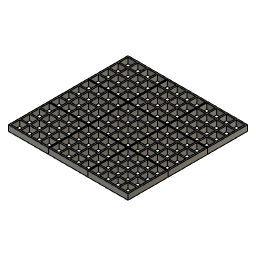
noycebru ws2812b 30 led per meter diffuser (Autodesk Fusion 360 design; units mm, degrees)
Autodesk Fusion 360 part; units mm, degrees
note: some values were not read from the file. Chosen so that the rebuilt part matches the saved one: which bodies a step acts on.
(part 1 of 2)
sketch "Sketch1" plane through (0, 0, 0) normal (0, 0, 1) x (1, 0, 0)
  line L0 (7.62, 66.04) -> (36.195, 66.04)
  line L1 (36.195, 66.04) -> (36.195, 37.465)
  line L2 (36.195, 37.465) -> (7.62, 37.465)
  line L3 (7.62, 37.465) -> (7.62, 66.04)
  line L4 (69.5325, 66.04) -> (69.5325, 37.465)
  line L5 (40.9575, 37.465) -> (40.9575, 66.04)
  line L6 (40.9575, 66.04) -> (69.5325, 66.04)
  line L7 (69.5325, 37.465) -> (40.9575, 37.465)
  line L8 (102.87, 66.04) -> (102.87, 37.465)
  line L9 (74.295, 37.465) -> (74.295, 66.04)
  line L10 (74.295, 66.04) -> (102.87, 66.04)
  line L11 (102.87, 37.465) -> (74.295, 37.465)
  line L12 (136.2075, 66.04) -> (136.2075, 37.465)
  line L13 (107.6325, 37.465) -> (107.6325, 66.04)
  line L14 (107.6325, 66.04) -> (136.2075, 66.04)
  line L15 (136.2075, 37.465) -> (107.6325, 37.465)
  line L16 (169.545, 66.04) -> (169.545, 37.465)
  line L17 (140.97, 37.465) -> (140.97, 66.04)
  line L18 (140.97, 66.04) -> (169.545, 66.04)
  line L19 (169.545, 37.465) -> (140.97, 37.465)
  line L20 (202.8825, 66.04) -> (202.8825, 37.465)
  line L21 (174.3075, 37.465) -> (174.3075, 66.04)
  line L22 (174.3075, 66.04) -> (202.8825, 66.04)
  line L23 (202.8825, 37.465) -> (174.3075, 37.465)
  line L24 (236.22, 66.04) -> (236.22, 37.465)
  line L25 (207.645, 37.465) -> (207.645, 66.04)
  line L26 (207.645, 66.04) -> (236.22, 66.04)
  line L27 (236.22, 37.465) -> (207.645, 37.465)
  line L28 (269.5575, 66.04) -> (269.5575, 37.465)
  line L29 (240.9825, 37.465) -> (240.9825, 66.04)
  line L30 (240.9825, 66.04) -> (269.5575, 66.04)
  line L31 (269.5575, 37.465) -> (240.9825, 37.465)
  line L32 (302.895, 66.04) -> (302.895, 37.465)
  line L33 (274.32, 37.465) -> (274.32, 66.04)
  line L34 (274.32, 66.04) -> (302.895, 66.04)
  line L35 (302.895, 37.465) -> (274.32, 37.465)
  line L36 (336.2325, 66.04) -> (336.2325, 37.465)
  line L37 (307.6575, 37.465) -> (307.6575, 66.04)
  line L38 (307.6575, 66.04) -> (336.2325, 66.04)
  line L39 (336.2325, 37.465) -> (307.6575, 37.465)
  line L40 (369.57, 66.04) -> (369.57, 37.465)
  line L41 (340.995, 37.465) -> (340.995, 66.04)
  line L42 (340.995, 66.04) -> (369.57, 66.04)
  line L43 (369.57, 37.465) -> (340.995, 37.465)
  line L44 (402.9075, 66.04) -> (402.9075, 37.465)
  line L45 (374.3325, 37.465) -> (374.3325, 66.04)
  line L46 (374.3325, 66.04) -> (402.9075, 66.04)
  line L47 (402.9075, 37.465) -> (374.3325, 37.465)
  line L48 (36.195, 99.3775) -> (36.195, 70.8025)
  line L49 (7.62, 70.8025) -> (7.62, 99.3775)
  line L50 (7.62, 99.3775) -> (36.195, 99.3775)
  line L51 (36.195, 70.8025) -> (7.62, 70.8025)
  line L52 (69.5325, 99.3775) -> (69.5325, 70.8025)
  line L53 (40.9575, 70.8025) -> (40.9575, 99.3775)
  line L54 (40.9575, 99.3775) -> (69.5325, 99.3775)
  line L55 (69.5325, 70.8025) -> (40.9575, 70.8025)
  line L56 (102.87, 99.3775) -> (102.87, 70.8025)
  line L57 (74.295, 70.8025) -> (74.295, 99.3775)
  line L58 (74.295, 99.3775) -> (102.87, 99.3775)
  line L59 (102.87, 70.8025) -> (74.295, 70.8025)
  line L60 (136.2075, 99.3775) -> (136.2075, 70.8025)
  line L61 (107.6325, 70.8025) -> (107.6325, 99.3775)
  line L62 (107.6325, 99.3775) -> (136.2075, 99.3775)
  line L63 (136.2075, 70.8025) -> (107.6325, 70.8025)
  line L64 (169.545, 99.3775) -> (169.545, 70.8025)
  line L65 (140.97, 70.8025) -> (140.97, 99.3775)
  line L66 (140.97, 99.3775) -> (169.545, 99.3775)
  line L67 (169.545, 70.8025) -> (140.97, 70.8025)
  line L68 (202.8825, 99.3775) -> (202.8825, 70.8025)
  line L69 (174.3075, 70.8025) -> (174.3075, 99.3775)
  line L70 (174.3075, 99.3775) -> (202.8825, 99.3775)
  line L71 (202.8825, 70.8025) -> (174.3075, 70.8025)
  line L72 (236.22, 99.3775) -> (236.22, 70.8025)
  line L73 (207.645, 70.8025) -> (207.645, 99.3775)
  line L74 (207.645, 99.3775) -> (236.22, 99.3775)
  line L75 (236.22, 70.8025) -> (207.645, 70.8025)
  line L76 (269.5575, 99.3775) -> (269.5575, 70.8025)
  line L77 (240.9825, 70.8025) -> (240.9825, 99.3775)
  line L78 (240.9825, 99.3775) -> (269.5575, 99.3775)
  line L79 (269.5575, 70.8025) -> (240.9825, 70.8025)
  line L80 (302.895, 99.3775) -> (302.895, 70.8025)
  line L81 (274.32, 70.8025) -> (274.32, 99.3775)
  line L82 (274.32, 99.3775) -> (302.895, 99.3775)
  line L83 (302.895, 70.8025) -> (274.32, 70.8025)
  line L84 (336.2325, 99.3775) -> (336.2325, 70.8025)
  line L85 (307.6575, 70.8025) -> (307.6575, 99.3775)
  line L86 (307.6575, 99.3775) -> (336.2325, 99.3775)
  line L87 (336.2325, 70.8025) -> (307.6575, 70.8025)
  line L88 (369.57, 99.3775) -> (369.57, 70.8025)
  line L89 (340.995, 70.8025) -> (340.995, 99.3775)
  line L90 (340.995, 99.3775) -> (369.57, 99.3775)
  line L91 (369.57, 70.8025) -> (340.995, 70.8025)
  line L92 (402.9075, 99.3775) -> (402.9075, 70.8025)
  line L93 (374.3325, 70.8025) -> (374.3325, 99.3775)
  line L94 (374.3325, 99.3775) -> (402.9075, 99.3775)
  line L95 (402.9075, 70.8025) -> (374.3325, 70.8025)
  line L96 (36.195, 132.715) -> (36.195, 104.14)
  line L97 (7.62, 104.14) -> (7.62, 132.715)
  line L98 (7.62, 132.715) -> (36.195, 132.715)
  line L99 (36.195, 104.14) -> (7.62, 104.14)
  line L100 (69.5325, 132.715) -> (69.5325, 104.14)
  line L101 (40.9575, 104.14) -> (40.9575, 132.715)
  line L102 (40.9575, 132.715) -> (69.5325, 132.715)
  line L103 (69.5325, 104.14) -> (40.9575, 104.14)
  line L104 (102.87, 132.715) -> (102.87, 104.14)
  line L105 (74.295, 104.14) -> (74.295, 132.715)
  line L106 (74.295, 132.715) -> (102.87, 132.715)
  line L107 (102.87, 104.14) -> (74.295, 104.14)
  line L108 (136.2075, 132.715) -> (136.2075, 104.14)
  line L109 (107.6325, 104.14) -> (107.6325, 132.715)
  line L110 (107.6325, 132.715) -> (136.2075, 132.715)
  line L111 (136.2075, 104.14) -> (107.6325, 104.14)
  line L112 (169.545, 132.715) -> (169.545, 104.14)
  line L113 (140.97, 104.14) -> (140.97, 132.715)
  line L114 (140.97, 132.715) -> (169.545, 132.715)
  line L115 (169.545, 104.14) -> (140.97, 104.14)
  line L116 (202.8825, 132.715) -> (202.8825, 104.14)
  line L117 (174.3075, 104.14) -> (174.3075, 132.715)
  line L118 (174.3075, 132.715) -> (202.8825, 132.715)
  line L119 (202.8825, 104.14) -> (174.3075, 104.14)
  line L120 (236.22, 132.715) -> (236.22, 104.14)
  line L121 (207.645, 104.14) -> (207.645, 132.715)
  line L122 (207.645, 132.715) -> (236.22, 132.715)
  line L123 (236.22, 104.14) -> (207.645, 104.14)
  line L124 (269.5575, 132.715) -> (269.5575, 104.14)
  line L125 (240.9825, 104.14) -> (240.9825, 132.715)
  line L126 (240.9825, 132.715) -> (269.5575, 132.715)
  line L127 (269.5575, 104.14) -> (240.9825, 104.14)
  line L128 (302.895, 132.715) -> (302.895, 104.14)
  line L129 (274.32, 104.14) -> (274.32, 132.715)
  line L130 (274.32, 132.715) -> (302.895, 132.715)
  line L131 (302.895, 104.14) -> (274.32, 104.14)
  line L132 (336.2325, 132.715) -> (336.2325, 104.14)
  line L133 (307.6575, 104.14) -> (307.6575, 132.715)
  line L134 (307.6575, 132.715) -> (336.2325, 132.715)
  line L135 (336.2325, 104.14) -> (307.6575, 104.14)
  line L136 (369.57, 132.715) -> (369.57, 104.14)
  line L137 (340.995, 104.14) -> (340.995, 132.715)
  line L138 (340.995, 132.715) -> (369.57, 132.715)
  line L139 (369.57, 104.14) -> (340.995, 104.14)
  line L140 (402.9075, 132.715) -> (402.9075, 104.14)
  line L141 (374.3325, 104.14) -> (374.3325, 132.715)
  line L142 (374.3325, 132.715) -> (402.9075, 132.715)
  line L143 (402.9075, 104.14) -> (374.3325, 104.14)
  line L144 (36.195, 166.0525) -> (36.195, 137.4775)
  line L145 (7.62, 137.4775) -> (7.62, 166.0525)
  line L146 (7.62, 166.0525) -> (36.195, 166.0525)
  line L147 (36.195, 137.4775) -> (7.62, 137.4775)
  line L148 (69.5325, 166.0525) -> (69.5325, 137.4775)
  line L149 (40.9575, 137.4775) -> (40.9575, 166.0525)
  line L150 (40.9575, 166.0525) -> (69.5325, 166.0525)
  line L151 (69.5325, 137.4775) -> (40.9575, 137.4775)
  line L152 (102.87, 166.0525) -> (102.87, 137.4775)
  line L153 (74.295, 137.4775) -> (74.295, 166.0525)
  line L154 (74.295, 166.0525) -> (102.87, 166.0525)
  line L155 (102.87, 137.4775) -> (74.295, 137.4775)
  line L156 (136.2075, 166.0525) -> (136.2075, 137.4775)
  line L157 (107.6325, 137.4775) -> (107.6325, 166.0525)
  line L158 (107.6325, 166.0525) -> (136.2075, 166.0525)
  line L159 (136.2075, 137.4775) -> (107.6325, 137.4775)
  line L160 (169.545, 166.0525) -> (169.545, 137.4775)
  line L161 (140.97, 137.4775) -> (140.97, 166.0525)
  line L162 (140.97, 166.0525) -> (169.545, 166.0525)
  line L163 (169.545, 137.4775) -> (140.97, 137.4775)
  line L164 (202.8825, 166.0525) -> (202.8825, 137.4775)
  line L165 (174.3075, 137.4775) -> (174.3075, 166.0525)
  line L166 (174.3075, 166.0525) -> (202.8825, 166.0525)
  line L167 (202.8825, 137.4775) -> (174.3075, 137.4775)
  line L168 (236.22, 166.0525) -> (236.22, 137.4775)
  line L169 (207.645, 137.4775) -> (207.645, 166.0525)
  line L170 (207.645, 166.0525) -> (236.22, 166.0525)
  line L171 (236.22, 137.4775) -> (207.645, 137.4775)
  line L172 (269.5575, 166.0525) -> (269.5575, 137.4775)
  line L173 (240.9825, 137.4775) -> (240.9825, 166.0525)
  line L174 (240.9825, 166.0525) -> (269.5575, 166.0525)
  line L175 (269.5575, 137.4775) -> (240.9825, 137.4775)
  line L176 (302.895, 166.0525) -> (302.895, 137.4775)
  line L177 (274.32, 137.4775) -> (274.32, 166.0525)
  line L178 (274.32, 166.0525) -> (302.895, 166.0525)
  line L179 (302.895, 137.4775) -> (274.32, 137.4775)
  line L180 (336.2325, 166.0525) -> (336.2325, 137.4775)
  line L181 (307.6575, 137.4775) -> (307.6575, 166.0525)
  line L182 (307.6575, 166.0525) -> (336.2325, 166.0525)
  line L183 (336.2325, 137.4775) -> (307.6575, 137.4775)
  line L184 (369.57, 166.0525) -> (369.57, 137.4775)
  line L185 (340.995, 137.4775) -> (340.995, 166.0525)
  line L186 (340.995, 166.0525) -> (369.57, 166.0525)
  line L187 (369.57, 137.4775) -> (340.995, 137.4775)
  line L188 (402.9075, 166.0525) -> (402.9075, 137.4775)
  line L189 (374.3325, 137.4775) -> (374.3325, 166.0525)
  line L190 (374.3325, 166.0525) -> (402.9075, 166.0525)
  line L191 (402.9075, 137.4775) -> (374.3325, 137.4775)
  line L192 (36.195, 199.39) -> (36.195, 170.815)
  line L193 (7.62, 170.815) -> (7.62, 199.39)
  line L194 (7.62, 199.39) -> (36.195, 199.39)
  line L195 (36.195, 170.815) -> (7.62, 170.815)
  line L196 (69.5325, 199.39) -> (69.5325, 170.815)
  line L197 (40.9575, 170.815) -> (40.9575, 199.39)
  line L198 (40.9575, 199.39) -> (69.5325, 199.39)
  line L199 (69.5325, 170.815) -> (40.9575, 170.815)
  line L200 (102.87, 199.39) -> (102.87, 170.815)
  line L201 (74.295, 170.815) -> (74.295, 199.39)
  line L202 (74.295, 199.39) -> (102.87, 199.39)
  line L203 (102.87, 170.815) -> (74.295, 170.815)
  line L204 (136.2075, 199.39) -> (136.2075, 170.815)
  line L205 (107.6325, 170.815) -> (107.6325, 199.39)
  line L206 (107.6325, 199.39) -> (136.2075, 199.39)
  line L207 (136.2075, 170.815) -> (107.6325, 170.815)
  line L208 (169.545, 199.39) -> (169.545, 170.815)
  line L209 (140.97, 170.815) -> (140.97, 199.39)
  line L210 (140.97, 199.39) -> (169.545, 199.39)
  line L211 (169.545, 170.815) -> (140.97, 170.815)
  line L212 (202.8825, 199.39) -> (202.8825, 170.815)
  line L213 (174.3075, 170.815) -> (174.3075, 199.39)
  line L214 (174.3075, 199.39) -> (202.8825, 199.39)
  line L215 (202.8825, 170.815) -> (174.3075, 170.815)
  line L216 (236.22, 199.39) -> (236.22, 170.815)
  line L217 (207.645, 170.815) -> (207.645, 199.39)
  line L218 (207.645, 199.39) -> (236.22, 199.39)
  line L219 (236.22, 170.815) -> (207.645, 170.815)
  line L220 (269.5575, 199.39) -> (269.5575, 170.815)
  line L221 (240.9825, 170.815) -> (240.9825, 199.39)
  line L222 (240.9825, 199.39) -> (269.5575, 199.39)
  line L223 (269.5575, 170.815) -> (240.9825, 170.815)
  line L224 (302.895, 199.39) -> (302.895, 170.815)
  line L225 (274.32, 170.815) -> (274.32, 199.39)
  line L226 (274.32, 199.39) -> (302.895, 199.39)
  line L227 (302.895, 170.815) -> (274.32, 170.815)
  line L228 (336.2325, 199.39) -> (336.2325, 170.815)
  line L229 (307.6575, 170.815) -> (307.6575, 199.39)
  line L230 (307.6575, 199.39) -> (336.2325, 199.39)
  line L231 (336.2325, 170.815) -> (307.6575, 170.815)
  line L232 (369.57, 199.39) -> (369.57, 170.815)
  line L233 (340.995, 170.815) -> (340.995, 199.39)
  line L234 (340.995, 199.39) -> (369.57, 199.39)
  line L235 (369.57, 170.815) -> (340.995, 170.815)
  line L236 (402.9075, 199.39) -> (402.9075, 170.815)
  line L237 (374.3325, 170.815) -> (374.3325, 199.39)
  line L238 (374.3325, 199.39) -> (402.9075, 199.39)
  line L239 (402.9075, 170.815) -> (374.3325, 170.815)
  line L240 (36.195, 232.7275) -> (36.195, 204.1525)
  line L241 (7.62, 204.1525) -> (7.62, 232.7275)
  line L242 (7.62, 232.7275) -> (36.195, 232.7275)
  line L243 (36.195, 204.1525) -> (7.62, 204.1525)
  line L244 (69.5325, 232.7275) -> (69.5325, 204.1525)
  line L245 (40.9575, 204.1525) -> (40.9575, 232.7275)
  line L246 (40.9575, 232.7275) -> (69.5325, 232.7275)
  line L247 (69.5325, 204.1525) -> (40.9575, 204.1525)
  line L248 (102.87, 232.7275) -> (102.87, 204.1525)
  line L249 (74.295, 204.1525) -> (74.295, 232.7275)
  line L250 (74.295, 232.7275) -> (102.87, 232.7275)
  line L251 (102.87, 204.1525) -> (74.295, 204.1525)
  line L252 (136.2075, 232.7275) -> (136.2075, 204.1525)
  line L253 (107.6325, 204.1525) -> (107.6325, 232.7275)
  line L254 (107.6325, 232.7275) -> (136.2075, 232.7275)
  line L255 (136.2075, 204.1525) -> (107.6325, 204.1525)
  line L256 (169.545, 232.7275) -> (169.545, 204.1525)
  line L257 (140.97, 204.1525) -> (140.97, 232.7275)
  line L258 (140.97, 232.7275) -> (169.545, 232.7275)
  line L259 (169.545, 204.1525) -> (140.97, 204.1525)
  line L260 (202.8825, 232.7275) -> (202.8825, 204.1525)
  line L261 (174.3075, 204.1525) -> (174.3075, 232.7275)
  line L262 (174.3075, 232.7275) -> (202.8825, 232.7275)
  line L263 (202.8825, 204.1525) -> (174.3075, 204.1525)
  line L264 (236.22, 232.7275) -> (236.22, 204.1525)
  line L265 (207.645, 204.1525) -> (207.645, 232.7275)
  line L266 (207.645, 232.7275) -> (236.22, 232.7275)
  line L267 (236.22, 204.1525) -> (207.645, 204.1525)
  line L268 (269.5575, 232.7275) -> (269.5575, 204.1525)
  line L269 (240.9825, 204.1525) -> (240.9825, 232.7275)
  line L270 (240.9825, 232.7275) -> (269.5575, 232.7275)
  line L271 (269.5575, 204.1525) -> (240.9825, 204.1525)
  line L272 (302.895, 232.7275) -> (302.895, 204.1525)
  line L273 (274.32, 204.1525) -> (274.32, 232.7275)
  line L274 (274.32, 232.7275) -> (302.895, 232.7275)
  line L275 (302.895, 204.1525) -> (274.32, 204.1525)
  line L276 (336.2325, 232.7275) -> (336.2325, 204.1525)
  line L277 (307.6575, 204.1525) -> (307.6575, 232.7275)
  line L278 (307.6575, 232.7275) -> (336.2325, 232.7275)
  line L279 (336.2325, 204.1525) -> (307.6575, 204.1525)
  line L280 (369.57, 232.7275) -> (369.57, 204.1525)
  line L281 (340.995, 204.1525) -> (340.995, 232.7275)
  line L282 (340.995, 232.7275) -> (369.57, 232.7275)
  line L283 (369.57, 204.1525) -> (340.995, 204.1525)
  line L284 (402.9075, 232.7275) -> (402.9075, 204.1525)
  line L285 (374.3325, 204.1525) -> (374.3325, 232.7275)
  line L286 (374.3325, 232.7275) -> (402.9075, 232.7275)
  line L287 (402.9075, 204.1525) -> (374.3325, 204.1525)
  line L288 (36.195, 266.065) -> (36.195, 237.49)
  line L289 (7.62, 237.49) -> (7.62, 266.065)
  line L290 (7.62, 266.065) -> (36.195, 266.065)
  line L291 (36.195, 237.49) -> (7.62, 237.49)
  line L292 (69.5325, 266.065) -> (69.5325, 237.49)
  line L293 (40.9575, 237.49) -> (40.9575, 266.065)
  line L294 (40.9575, 266.065) -> (69.5325, 266.065)
  line L295 (69.5325, 237.49) -> (40.9575, 237.49)
  line L296 (102.87, 266.065) -> (102.87, 237.49)
  line L297 (74.295, 237.49) -> (74.295, 266.065)
  line L298 (74.295, 266.065) -> (102.87, 266.065)
  line L299 (102.87, 237.49) -> (74.295, 237.49)
  line L300 (136.2075, 266.065) -> (136.2075, 237.49)
  line L301 (107.6325, 237.49) -> (107.6325, 266.065)
  line L302 (107.6325, 266.065) -> (136.2075, 266.065)
  line L303 (136.2075, 237.49) -> (107.6325, 237.49)
  line L304 (169.545, 266.065) -> (169.545, 237.49)
  line L305 (140.97, 237.49) -> (140.97, 266.065)
  line L306 (140.97, 266.065) -> (169.545, 266.065)
  line L307 (169.545, 237.49) -> (140.97, 237.49)
  line L308 (202.8825, 266.065) -> (202.8825, 237.49)
  line L309 (174.3075, 237.49) -> (174.3075, 266.065)
  line L310 (174.3075, 266.065) -> (202.8825, 266.065)
  line L311 (202.8825, 237.49) -> (174.3075, 237.49)
  line L312 (236.22, 266.065) -> (236.22, 237.49)
  line L313 (207.645, 237.49) -> (207.645, 266.065)
  line L314 (207.645, 266.065) -> (236.22, 266.065)
  line L315 (236.22, 237.49) -> (207.645, 237.49)
  line L316 (269.5575, 266.065) -> (269.5575, 237.49)
  line L317 (240.9825, 237.49) -> (240.9825, 266.065)
  line L318 (240.9825, 266.065) -> (269.5575, 266.065)
  line L319 (269.5575, 237.49) -> (240.9825, 237.49)
  line L320 (302.895, 266.065) -> (302.895, 237.49)
  line L321 (274.32, 237.49) -> (274.32, 266.065)
  line L322 (274.32, 266.065) -> (302.895, 266.065)
  line L323 (302.895, 237.49) -> (274.32, 237.49)
  line L324 (336.2325, 266.065) -> (336.2325, 237.49)
  line L325 (307.6575, 237.49) -> (307.6575, 266.065)
  line L326 (307.6575, 266.065) -> (336.2325, 266.065)
  line L327 (336.2325, 237.49) -> (307.6575, 237.49)
  line L328 (369.57, 266.065) -> (369.57, 237.49)
  line L329 (340.995, 237.49) -> (340.995, 266.065)
  line L330 (340.995, 266.065) -> (369.57, 266.065)
  line L331 (369.57, 237.49) -> (340.995, 237.49)
  line L332 (402.9075, 266.065) -> (402.9075, 237.49)
  line L333 (374.3325, 237.49) -> (374.3325, 266.065)
  line L334 (374.3325, 266.065) -> (402.9075, 266.065)
  line L335 (402.9075, 237.49) -> (374.3325, 237.49)
  line L336 (36.195, 299.4025) -> (36.195, 270.8275)
  line L337 (7.62, 270.8275) -> (7.62, 299.4025)
  line L338 (7.62, 299.4025) -> (36.195, 299.4025)
  line L339 (36.195, 270.8275) -> (7.62, 270.8275)
  line L340 (69.5325, 299.4025) -> (69.5325, 270.8275)
  line L341 (40.9575, 270.8275) -> (40.9575, 299.4025)
  line L342 (40.9575, 299.4025) -> (69.5325, 299.4025)
  line L343 (69.5325, 270.8275) -> (40.9575, 270.8275)
  line L344 (102.87, 299.4025) -> (102.87, 270.8275)
  line L345 (74.295, 270.8275) -> (74.295, 299.4025)
  line L346 (74.295, 299.4025) -> (102.87, 299.4025)
  line L347 (102.87, 270.8275) -> (74.295, 270.8275)
  line L348 (136.2075, 299.4025) -> (136.2075, 270.8275)
  line L349 (107.6325, 270.8275) -> (107.6325, 299.4025)
  line L350 (107.6325, 299.4025) -> (136.2075, 299.4025)
  line L351 (136.2075, 270.8275) -> (107.6325, 270.8275)
  line L352 (169.545, 299.4025) -> (169.545, 270.8275)
  line L353 (140.97, 270.8275) -> (140.97, 299.4025)
  line L354 (140.97, 299.4025) -> (169.545, 299.4025)
  line L355 (169.545, 270.8275) -> (140.97, 270.8275)
  line L356 (202.8825, 299.4025) -> (202.8825, 270.8275)
  line L357 (174.3075, 270.8275) -> (174.3075, 299.4025)
  line L358 (174.3075, 299.4025) -> (202.8825, 299.4025)
  line L359 (202.8825, 270.8275) -> (174.3075, 270.8275)
  line L360 (236.22, 299.4025) -> (236.22, 270.8275)
  line L361 (207.645, 270.8275) -> (207.645, 299.4025)
  line L362 (207.645, 299.4025) -> (236.22, 299.4025)
  line L363 (236.22, 270.8275) -> (207.645, 270.8275)
  line L364 (269.5575, 299.4025) -> (269.5575, 270.8275)
  line L365 (240.9825, 270.8275) -> (240.9825, 299.4025)
  line L366 (240.9825, 299.4025) -> (269.5575, 299.4025)
  line L367 (269.5575, 270.8275) -> (240.9825, 270.8275)
  line L368 (302.895, 299.4025) -> (302.895, 270.8275)
  line L369 (274.32, 270.8275) -> (274.32, 299.4025)
  line L370 (274.32, 299.4025) -> (302.895, 299.4025)
  line L371 (302.895, 270.8275) -> (274.32, 270.8275)
  line L372 (336.2325, 299.4025) -> (336.2325, 270.8275)
  line L373 (307.6575, 270.8275) -> (307.6575, 299.4025)
  line L374 (307.6575, 299.4025) -> (336.2325, 299.4025)
  line L375 (336.2325, 270.8275) -> (307.6575, 270.8275)
  line L376 (369.57, 299.4025) -> (369.57, 270.8275)
  line L377 (340.995, 270.8275) -> (340.995, 299.4025)
  line L378 (340.995, 299.4025) -> (369.57, 299.4025)
  line L379 (369.57, 270.8275) -> (340.995, 270.8275)
  line L380 (402.9075, 299.4025) -> (402.9075, 270.8275)
  line L381 (374.3325, 270.8275) -> (374.3325, 299.4025)
  line L382 (374.3325, 299.4025) -> (402.9075, 299.4025)
  line L383 (402.9075, 270.8275) -> (374.3325, 270.8275)
  line L384 (36.195, 332.74) -> (36.195, 304.165)
  line L385 (7.62, 304.165) -> (7.62, 332.74)
  line L386 (7.62, 332.74) -> (36.195, 332.74)
  line L387 (36.195, 304.165) -> (7.62, 304.165)
  line L388 (69.5325, 332.74) -> (69.5325, 304.165)
  line L389 (40.9575, 304.165) -> (40.9575, 332.74)
  line L390 (40.9575, 332.74) -> (69.5325, 332.74)
  line L391 (69.5325, 304.165) -> (40.9575, 304.165)
  line L392 (102.87, 332.74) -> (102.87, 304.165)
  line L393 (74.295, 304.165) -> (74.295, 332.74)
  line L394 (74.295, 332.74) -> (102.87, 332.74)
  line L395 (102.87, 304.165) -> (74.295, 304.165)
  line L396 (136.2075, 332.74) -> (136.2075, 304.165)
  line L397 (107.6325, 304.165) -> (107.6325, 332.74)
  line L398 (107.6325, 332.74) -> (136.2075, 332.74)
  line L399 (136.2075, 304.165) -> (107.6325, 304.165)
  line L400 (169.545, 332.74) -> (169.545, 304.165)
  line L401 (140.97, 304.165) -> (140.97, 332.74)
  line L402 (140.97, 332.74) -> (169.545, 332.74)
  line L403 (169.545, 304.165) -> (140.97, 304.165)
  line L404 (202.8825, 332.74) -> (202.8825, 304.165)
  line L405 (174.3075, 304.165) -> (174.3075, 332.74)
  line L406 (174.3075, 332.74) -> (202.8825, 332.74)
  line L407 (202.8825, 304.165) -> (174.3075, 304.165)
  line L408 (236.22, 332.74) -> (236.22, 304.165)
  line L409 (207.645, 304.165) -> (207.645, 332.74)
  line L410 (207.645, 332.74) -> (236.22, 332.74)
  line L411 (236.22, 304.165) -> (207.645, 304.165)
  line L412 (269.5575, 332.74) -> (269.5575, 304.165)
  line L413 (240.9825, 304.165) -> (240.9825, 332.74)
  line L414 (240.9825, 332.74) -> (269.5575, 332.74)
  line L415 (269.5575, 304.165) -> (240.9825, 304.165)
  line L416 (302.895, 332.74) -> (302.895, 304.165)
  line L417 (274.32, 304.165) -> (274.32, 332.74)
  line L418 (274.32, 332.74) -> (302.895, 332.74)
  line L419 (302.895, 304.165) -> (274.32, 304.165)
  line L420 (336.2325, 332.74) -> (336.2325, 304.165)
  line L421 (307.6575, 304.165) -> (307.6575, 332.74)
  line L422 (307.6575, 332.74) -> (336.2325, 332.74)
  line L423 (336.2325, 304.165) -> (307.6575, 304.165)
  line L424 (369.57, 332.74) -> (369.57, 304.165)
  line L425 (340.995, 304.165) -> (340.995, 332.74)
  line L426 (340.995, 332.74) -> (369.57, 332.74)
  line L427 (369.57, 304.165) -> (340.995, 304.165)
  line L428 (402.9075, 332.74) -> (402.9075, 304.165)
  line L429 (374.3325, 304.165) -> (374.3325, 332.74)
  line L430 (374.3325, 332.74) -> (402.9075, 332.74)
  line L431 (402.9075, 304.165) -> (374.3325, 304.165)
  line L432 (36.195, 366.0775) -> (36.195, 337.5025)
  line L433 (7.62, 337.5025) -> (7.62, 366.0775)
  line L434 (7.62, 366.0775) -> (36.195, 366.0775)
  line L435 (36.195, 337.5025) -> (7.62, 337.5025)
  line L436 (69.5325, 366.0775) -> (69.5325, 337.5025)
  line L437 (40.9575, 337.5025) -> (40.9575, 366.0775)
  line L438 (40.9575, 366.0775) -> (69.5325, 366.0775)
  line L439 (69.5325, 337.5025) -> (40.9575, 337.5025)
  line L440 (102.87, 366.0775) -> (102.87, 337.5025)
  line L441 (74.295, 337.5025) -> (74.295, 366.0775)
  line L442 (74.295, 366.0775) -> (102.87, 366.0775)
  line L443 (102.87, 337.5025) -> (74.295, 337.5025)
  line L444 (136.2075, 366.0775) -> (136.2075, 337.5025)
  line L445 (107.6325, 337.5025) -> (107.6325, 366.0775)
  line L446 (107.6325, 366.0775) -> (136.2075, 366.0775)
  line L447 (136.2075, 337.5025) -> (107.6325, 337.5025)
  line L448 (169.545, 366.0775) -> (169.545, 337.5025)
  line L449 (140.97, 337.5025) -> (140.97, 366.0775)
  line L450 (140.97, 366.0775) -> (169.545, 366.0775)
  line L451 (169.545, 337.5025) -> (140.97, 337.5025)
  line L452 (202.8825, 366.0775) -> (202.8825, 337.5025)
  line L453 (174.3075, 337.5025) -> (174.3075, 366.0775)
  line L454 (174.3075, 366.0775) -> (202.8825, 366.0775)
  line L455 (202.8825, 337.5025) -> (174.3075, 337.5025)
  line L456 (236.22, 366.0775) -> (236.22, 337.5025)
  line L457 (207.645, 337.5025) -> (207.645, 366.0775)
  line L458 (207.645, 366.0775) -> (236.22, 366.0775)
  line L459 (236.22, 337.5025) -> (207.645, 337.5025)
  line L460 (269.5575, 366.0775) -> (269.5575, 337.5025)
  line L461 (240.9825, 337.5025) -> (240.9825, 366.0775)
  line L462 (240.9825, 366.0775) -> (269.5575, 366.0775)
  line L463 (269.5575, 337.5025) -> (240.9825, 337.5025)
  line L464 (302.895, 366.0775) -> (302.895, 337.5025)
  line L465 (274.32, 337.5025) -> (274.32, 366.0775)
  line L466 (274.32, 366.0775) -> (302.895, 366.0775)
  line L467 (302.895, 337.5025) -> (274.32, 337.5025)
  line L468 (336.2325, 366.0775) -> (336.2325, 337.5025)
  line L469 (307.6575, 337.5025) -> (307.6575, 366.0775)
  line L470 (307.6575, 366.0775) -> (336.2325, 366.0775)
  line L471 (336.2325, 337.5025) -> (307.6575, 337.5025)
  line L472 (369.57, 366.0775) -> (369.57, 337.5025)
  line L473 (340.995, 337.5025) -> (340.995, 366.0775)
  line L474 (340.995, 366.0775) -> (369.57, 366.0775)
  line L475 (369.57, 337.5025) -> (340.995, 337.5025)
  line L476 (402.9075, 366.0775) -> (402.9075, 337.5025)
  line L477 (374.3325, 337.5025) -> (374.3325, 366.0775)
  line L478 (374.3325, 366.0775) -> (402.9075, 366.0775)
  line L479 (402.9075, 337.5025) -> (374.3325, 337.5025)
  line L480 (36.195, 399.415) -> (36.195, 370.84)
  line L481 (7.62, 370.84) -> (7.62, 399.415)
  line L482 (7.62, 399.415) -> (36.195, 399.415)
  line L483 (36.195, 370.84) -> (7.62, 370.84)
  line L484 (69.5325, 399.415) -> (69.5325, 370.84)
  line L485 (40.9575, 370.84) -> (40.9575, 399.415)
  line L486 (40.9575, 399.415) -> (69.5325, 399.415)
  line L487 (69.5325, 370.84) -> (40.9575, 370.84)
  line L488 (102.87, 399.415) -> (102.87, 370.84)
  line L489 (74.295, 370.84) -> (74.295, 399.415)
  line L490 (74.295, 399.415) -> (102.87, 399.415)
  line L491 (102.87, 370.84) -> (74.295, 370.84)
  line L492 (136.2075, 399.415) -> (136.2075, 370.84)
  line L493 (107.6325, 370.84) -> (107.6325, 399.415)
  line L494 (107.6325, 399.415) -> (136.2075, 399.415)
  line L495 (136.2075, 370.84) -> (107.6325, 370.84)
  line L496 (169.545, 399.415) -> (169.545, 370.84)
  line L497 (140.97, 370.84) -> (140.97, 399.415)
  line L498 (140.97, 399.415) -> (169.545, 399.415)
  line L499 (169.545, 370.84) -> (140.97, 370.84)
  line L500 (202.8825, 399.415) -> (202.8825, 370.84)
  line L501 (174.3075, 370.84) -> (174.3075, 399.415)
  line L502 (174.3075, 399.415) -> (202.8825, 399.415)
  line L503 (202.8825, 370.84) -> (174.3075, 370.84)
  line L504 (236.22, 399.415) -> (236.22, 370.84)
  line L505 (207.645, 370.84) -> (207.645, 399.415)
  line L506 (207.645, 399.415) -> (236.22, 399.415)
  line L507 (236.22, 370.84) -> (207.645, 370.84)
  line L508 (269.5575, 399.415) -> (269.5575, 370.84)
  line L509 (240.9825, 370.84) -> (240.9825, 399.415)
  line L510 (240.9825, 399.415) -> (269.5575, 399.415)
  line L511 (269.5575, 370.84) -> (240.9825, 370.84)
  line L512 (302.895, 399.415) -> (302.895, 370.84)
  line L513 (274.32, 370.84) -> (274.32, 399.415)
  line L514 (274.32, 399.415) -> (302.895, 399.415)
  line L515 (302.895, 370.84) -> (274.32, 370.84)
  line L516 (336.2325, 399.415) -> (336.2325, 370.84)
  line L517 (307.6575, 370.84) -> (307.6575, 399.415)
  line L518 (307.6575, 399.415) -> (336.2325, 399.415)
  line L519 (336.2325, 370.84) -> (307.6575, 370.84)
  line L520 (369.57, 399.415) -> (369.57, 370.84)
  line L521 (340.995, 370.84) -> (340.995, 399.415)
  line L522 (340.995, 399.415) -> (369.57, 399.415)
  line L523 (369.57, 370.84) -> (340.995, 370.84)
  line L524 (402.9075, 399.415) -> (402.9075, 370.84)
  line L525 (374.3325, 370.84) -> (374.3325, 399.415)
  line L526 (374.3325, 399.415) -> (402.9075, 399.415)
  line L527 (402.9075, 370.84) -> (374.3325, 370.84)
  line L528 (36.195, 432.7525) -> (36.195, 404.1775)
  line L529 (7.62, 404.1775) -> (7.62, 432.7525)
  line L530 (7.62, 432.7525) -> (36.195, 432.7525)
  line L531 (36.195, 404.1775) -> (7.62, 404.1775)
  line L532 (69.5325, 432.7525) -> (69.5325, 404.1775)
  line L533 (40.9575, 404.1775) -> (40.9575, 432.7525)
  line L534 (40.9575, 432.7525) -> (69.5325, 432.7525)
  line L535 (69.5325, 404.1775) -> (40.9575, 404.1775)
  line L536 (102.87, 432.7525) -> (102.87, 404.1775)
  line L537 (74.295, 404.1775) -> (74.295, 432.7525)
  line L538 (74.295, 432.7525) -> (102.87, 432.7525)
  line L539 (102.87, 404.1775) -> (74.295, 404.1775)
  line L540 (136.2075, 432.7525) -> (136.2075, 404.1775)
  line L541 (107.6325, 404.1775) -> (107.6325, 432.7525)
  line L542 (107.6325, 432.7525) -> (136.2075, 432.7525)
  line L543 (136.2075, 404.1775) -> (107.6325, 404.1775)
  line L544 (169.545, 432.7525) -> (169.545, 404.1775)
  line L545 (140.97, 404.1775) -> (140.97, 432.7525)
  line L546 (140.97, 432.7525) -> (169.545, 432.7525)
  line L547 (169.545, 404.1775) -> (140.97, 404.1775)
  line L548 (202.8825, 432.7525) -> (202.8825, 404.1775)
  line L549 (174.3075, 404.1775) -> (174.3075, 432.7525)
  line L550 (174.3075, 432.7525) -> (202.8825, 432.7525)
  line L551 (202.8825, 404.1775) -> (174.3075, 404.1775)
  line L552 (236.22, 432.7525) -> (236.22, 404.1775)
  line L553 (207.645, 404.1775) -> (207.645, 432.7525)
  line L554 (207.645, 432.7525) -> (236.22, 432.7525)
  line L555 (236.22, 404.1775) -> (207.645, 404.1775)
  line L556 (269.5575, 432.7525) -> (269.5575, 404.1775)
  line L557 (240.9825, 404.1775) -> (240.9825, 432.7525)
  line L558 (240.9825, 432.7525) -> (269.5575, 432.7525)
  line L559 (269.5575, 404.1775) -> (240.9825, 404.1775)
  line L560 (302.895, 432.7525) -> (302.895, 404.1775)
  line L561 (274.32, 404.1775) -> (274.32, 432.7525)
  line L562 (274.32, 432.7525) -> (302.895, 432.7525)
  line L563 (302.895, 404.1775) -> (274.32, 404.1775)
  line L564 (336.2325, 432.7525) -> (336.2325, 404.1775)
  line L565 (307.6575, 404.1775) -> (307.6575, 432.7525)
  line L566 (307.6575, 432.7525) -> (336.2325, 432.7525)
  line L567 (336.2325, 404.1775) -> (307.6575, 404.1775)
  line L568 (369.57, 432.7525) -> (369.57, 404.1775)
  line L569 (340.995, 404.1775) -> (340.995, 432.7525)
  line L570 (340.995, 432.7525) -> (369.57, 432.7525)
  line L571 (369.57, 404.1775) -> (340.995, 404.1775)
  line L572 (402.9075, 432.7525) -> (402.9075, 404.1775)
  line L573 (374.3325, 404.1775) -> (374.3325, 432.7525)
  line L574 (374.3325, 432.7525) -> (402.9075, 432.7525)
  line L575 (402.9075, 404.1775) -> (374.3325, 404.1775)
  line L576 (36.195, 399.415) -> (7.62, 399.415)
  line L577 (2.8575, 399.415) -> (2.8575, 437.515)
  line L578 (2.8575, 437.515) -> (40.9575, 437.515)
  line L579 (40.9575, 432.7525) -> (40.9575, 404.1775)
  line L580 (402.9075, 399.415) -> (374.3325, 399.415)
  line L581 (369.57, 404.1775) -> (369.57, 432.7525)
  line L582 (369.57, 437.515) -> (407.67, 437.515)
  line L583 (407.67, 437.515) -> (407.67, 399.415)
  line L584 (40.9575, 437.515) -> (369.57, 437.515)
  line L585 (369.57, 432.7525) -> (40.9575, 432.7525)
  line L586 (407.67, 32.7025) -> (369.57, 32.7025)
  line L587 (374.3325, 70.8025) -> (402.9075, 70.8025)
  line L588 (407.67, 70.8025) -> (407.67, 32.7025)
  line L589 (40.9575, 32.7025) -> (2.8575, 32.7025)
  line L590 (2.8575, 32.7025) -> (2.8575, 70.8025)
  line L591 (7.62, 70.8025) -> (36.195, 70.8025)
  line L592 (40.9575, 66.04) -> (40.9575, 37.465)
  line L593 (7.62, 399.415) -> (7.62, 70.8025)
  line L594 (2.8575, 70.8025) -> (2.8575, 399.415)
  line L595 (402.9075, 399.415) -> (402.9075, 70.8025)
  line L596 (407.67, 70.8025) -> (407.67, 399.415)
  line L597 (369.57, 32.7025) -> (40.9575, 32.7025)
  line L598 (40.9575, 37.465) -> (369.57, 37.465)
  dimension "d1" = 28.575
  dimension "d2" = 28.575
  dimension "d5" = 33.3375
  dimension "d6" = 33.3375
  constraint horizontal L0
  constraint vertical L1
  constraint horizontal L2
  constraint vertical L3
  constraint horizontal L584
  constraint horizontal L585
  constraint parallel L531 L576
  constraint parallel L529 L577
  constraint parallel L530 L578
  constraint parallel L528 L579
  constraint parallel L575 L580
  constraint parallel L573 L581
  constraint parallel L574 L582
  constraint parallel L572 L583
  constraint vertical L593
  constraint vertical L594
  constraint vertical L595
  constraint vertical L596
  constraint horizontal L597
  constraint horizontal L598
  constraint parallel L2 L589
  constraint parallel L3 L590
  constraint parallel L0 L591
  constraint parallel L1 L592
  constraint parallel L47 L586
  constraint parallel L46 L587
  constraint parallel L44 L588
  measures "d1" distance of L0.start L2.end
  measures "d2" distance of L0.start L0.end
extrude "Extrude1" add sketch "Sketch1" along normal blind 19.05 makes body 1
sketch "Sketch2" plane through (0, 0, 19.05) normal (0, 0, 1) x (-1, 0, 0)
  line L0 (-302.895, -132.715) -> (-302.895, -104.14)
  line L1 (-302.895, -104.14) -> (-274.32, -104.14)
  line L2 (-274.32, -104.14) -> (-274.32, -132.715)
  line L3 (-274.32, -132.715) -> (-302.895, -132.715)
  line L4 (-336.2325, -132.715) -> (-336.2325, -104.14)
  line L5 (-336.2325, -104.14) -> (-307.6575, -104.14)
  line L6 (-307.6575, -104.14) -> (-307.6575, -132.715)
  line L7 (-307.6575, -132.715) -> (-336.2325, -132.715)
  line L8 (-369.57, -132.715) -> (-369.57, -104.14)
  line L9 (-369.57, -104.14) -> (-340.995, -104.14)
  line L10 (-340.995, -104.14) -> (-340.995, -132.715)
  line L11 (-340.995, -132.715) -> (-369.57, -132.715)
  line L12 (-69.5325, -166.0525) -> (-69.5325, -137.4775)
  line L13 (-69.5325, -137.4775) -> (-40.9575, -137.4775)
  line L14 (-40.9575, -137.4775) -> (-40.9575, -166.0525)
  line L15 (-40.9575, -166.0525) -> (-69.5325, -166.0525)
  line L16 (-102.87, -166.0525) -> (-102.87, -137.4775)
  line L17 (-102.87, -137.4775) -> (-74.295, -137.4775)
  line L18 (-74.295, -137.4775) -> (-74.295, -166.0525)
  line L19 (-74.295, -166.0525) -> (-102.87, -166.0525)
  line L20 (-136.2075, -166.0525) -> (-136.2075, -137.4775)
  line L21 (-136.2075, -137.4775) -> (-107.6325, -137.4775)
  line L22 (-107.6325, -137.4775) -> (-107.6325, -166.0525)
  line L23 (-107.6325, -166.0525) -> (-136.2075, -166.0525)
  line L24 (-169.545, -166.0525) -> (-169.545, -137.4775)
  line L25 (-169.545, -137.4775) -> (-140.97, -137.4775)
  line L26 (-140.97, -137.4775) -> (-140.97, -166.0525)
  line L27 (-140.97, -166.0525) -> (-169.545, -166.0525)
  line L28 (-202.8825, -166.0525) -> (-202.8825, -137.4775)
  line L29 (-202.8825, -137.4775) -> (-174.3075, -137.4775)
  line L30 (-174.3075, -137.4775) -> (-174.3075, -166.0525)
  line L31 (-174.3075, -166.0525) -> (-202.8825, -166.0525)
  line L32 (-236.22, -166.0525) -> (-236.22, -137.4775)
  line L33 (-236.22, -137.4775) -> (-207.645, -137.4775)
  line L34 (-207.645, -137.4775) -> (-207.645, -166.0525)
  line L35 (-207.645, -166.0525) -> (-236.22, -166.0525)
  line L36 (-269.5575, -166.0525) -> (-269.5575, -137.4775)
  line L37 (-269.5575, -137.4775) -> (-240.9825, -137.4775)
  line L38 (-240.9825, -137.4775) -> (-240.9825, -166.0525)
  line L39 (-240.9825, -166.0525) -> (-269.5575, -166.0525)
  line L40 (-302.895, -166.0525) -> (-302.895, -137.4775)
  line L41 (-302.895, -137.4775) -> (-274.32, -137.4775)
  line L42 (-274.32, -137.4775) -> (-274.32, -166.0525)
  line L43 (-274.32, -166.0525) -> (-302.895, -166.0525)
  line L44 (-336.2325, -166.0525) -> (-336.2325, -137.4775)
  line L45 (-336.2325, -137.4775) -> (-307.6575, -137.4775)
  line L46 (-307.6575, -137.4775) -> (-307.6575, -166.0525)
  line L47 (-307.6575, -166.0525) -> (-336.2325, -166.0525)
  line L48 (-369.57, -166.0525) -> (-369.57, -137.4775)
  line L49 (-369.57, -137.4775) -> (-340.995, -137.4775)
  line L50 (-340.995, -137.4775) -> (-340.995, -166.0525)
  line L51 (-340.995, -166.0525) -> (-369.57, -166.0525)
  line L52 (-69.5325, -199.39) -> (-69.5325, -170.815)
  line L53 (-69.5325, -170.815) -> (-40.9575, -170.815)
  line L54 (-40.9575, -170.815) -> (-40.9575, -199.39)
  line L55 (-40.9575, -199.39) -> (-69.5325, -199.39)
  line L56 (-102.87, -199.39) -> (-102.87, -170.815)
  line L57 (-102.87, -170.815) -> (-74.295, -170.815)
  line L58 (-74.295, -170.815) -> (-74.295, -199.39)
  line L59 (-74.295, -199.39) -> (-102.87, -199.39)
  line L60 (-136.2075, -199.39) -> (-136.2075, -170.815)
  line L61 (-136.2075, -170.815) -> (-107.6325, -170.815)
  line L62 (-107.6325, -170.815) -> (-107.6325, -199.39)
  line L63 (-107.6325, -199.39) -> (-136.2075, -199.39)
  line L64 (-169.545, -199.39) -> (-169.545, -170.815)
  line L65 (-169.545, -170.815) -> (-140.97, -170.815)
  line L66 (-140.97, -170.815) -> (-140.97, -199.39)
  line L67 (-140.97, -199.39) -> (-169.545, -199.39)
  line L68 (-202.8825, -199.39) -> (-202.8825, -170.815)
  line L69 (-202.8825, -170.815) -> (-174.3075, -170.815)
  line L70 (-174.3075, -170.815) -> (-174.3075, -199.39)
  line L71 (-174.3075, -199.39) -> (-202.8825, -199.39)
  line L72 (-236.22, -199.39) -> (-236.22, -170.815)
  line L73 (-236.22, -170.815) -> (-207.645, -170.815)
  line L74 (-207.645, -170.815) -> (-207.645, -199.39)
  line L75 (-207.645, -199.39) -> (-236.22, -199.39)
  line L76 (-269.5575, -199.39) -> (-269.5575, -170.815)
  line L77 (-269.5575, -170.815) -> (-240.9825, -170.815)
  line L78 (-240.9825, -170.815) -> (-240.9825, -199.39)
  line L79 (-240.9825, -199.39) -> (-269.5575, -199.39)
  line L80 (-302.895, -199.39) -> (-302.895, -170.815)
  line L81 (-302.895, -170.815) -> (-274.32, -170.815)
  line L82 (-274.32, -170.815) -> (-274.32, -199.39)
  line L83 (-274.32, -199.39) -> (-302.895, -199.39)
  line L84 (-336.2325, -199.39) -> (-336.2325, -170.815)
  line L85 (-336.2325, -170.815) -> (-307.6575, -170.815)
  line L86 (-307.6575, -170.815) -> (-307.6575, -199.39)
  line L87 (-307.6575, -199.39) -> (-336.2325, -199.39)
  line L88 (-369.57, -199.39) -> (-369.57, -170.815)
  line L89 (-369.57, -170.815) -> (-340.995, -170.815)
  line L90 (-340.995, -170.815) -> (-340.995, -199.39)
  line L91 (-340.995, -199.39) -> (-369.57, -199.39)
  line L92 (-69.5325, -232.7275) -> (-69.5325, -204.1525)
  line L93 (-69.5325, -204.1525) -> (-40.9575, -204.1525)
  line L94 (-40.9575, -204.1525) -> (-40.9575, -232.7275)
  line L95 (-40.9575, -232.7275) -> (-69.5325, -232.7275)
  line L96 (-102.87, -232.7275) -> (-102.87, -204.1525)
  line L97 (-102.87, -204.1525) -> (-74.295, -204.1525)
  line L98 (-74.295, -204.1525) -> (-74.295, -232.7275)
  line L99 (-74.295, -232.7275) -> (-102.87, -232.7275)
  line L100 (-136.2075, -232.7275) -> (-136.2075, -204.1525)
  line L101 (-136.2075, -204.1525) -> (-107.6325, -204.1525)
  line L102 (-107.6325, -204.1525) -> (-107.6325, -232.7275)
  line L103 (-107.6325, -232.7275) -> (-136.2075, -232.7275)
  line L104 (-169.545, -232.7275) -> (-169.545, -204.1525)
  line L105 (-169.545, -204.1525) -> (-140.97, -204.1525)
  line L106 (-140.97, -204.1525) -> (-140.97, -232.7275)
  line L107 (-140.97, -232.7275) -> (-169.545, -232.7275)
  line L108 (-202.8825, -232.7275) -> (-202.8825, -204.1525)
  line L109 (-202.8825, -204.1525) -> (-174.3075, -204.1525)
  line L110 (-174.3075, -204.1525) -> (-174.3075, -232.7275)
  line L111 (-174.3075, -232.7275) -> (-202.8825, -232.7275)
  line L112 (-236.22, -232.7275) -> (-236.22, -204.1525)
  line L113 (-236.22, -204.1525) -> (-207.645, -204.1525)
  line L114 (-207.645, -204.1525) -> (-207.645, -232.7275)
  line L115 (-207.645, -232.7275) -> (-236.22, -232.7275)
  line L116 (-269.5575, -232.7275) -> (-269.5575, -204.1525)
  line L117 (-269.5575, -204.1525) -> (-240.9825, -204.1525)
  line L118 (-240.9825, -204.1525) -> (-240.9825, -232.7275)
  line L119 (-240.9825, -232.7275) -> (-269.5575, -232.7275)
  line L120 (-302.895, -232.7275) -> (-302.895, -204.1525)
  line L121 (-302.895, -204.1525) -> (-274.32, -204.1525)
  line L122 (-274.32, -204.1525) -> (-274.32, -232.7275)
  line L123 (-274.32, -232.7275) -> (-302.895, -232.7275)
  line L124 (-336.2325, -232.7275) -> (-336.2325, -204.1525)
  line L125 (-336.2325, -204.1525) -> (-307.6575, -204.1525)
  line L126 (-307.6575, -204.1525) -> (-307.6575, -232.7275)
  line L127 (-307.6575, -232.7275) -> (-336.2325, -232.7275)
  line L128 (-369.57, -232.7275) -> (-369.57, -204.1525)
  line L129 (-369.57, -204.1525) -> (-340.995, -204.1525)
  line L130 (-340.995, -204.1525) -> (-340.995, -232.7275)
  line L131 (-340.995, -232.7275) -> (-369.57, -232.7275)
  line L132 (-207.645, -432.7525) -> (-236.22, -432.7525)
  line L133 (-236.22, -432.7525) -> (-236.22, -404.1775)
  line L134 (-236.22, -404.1775) -> (-207.645, -404.1775)
  line L135 (-207.645, -404.1775) -> (-207.645, -432.7525)
  line L136 (-174.3075, -432.7525) -> (-202.8825, -432.7525)
  line L137 (-202.8825, -432.7525) -> (-202.8825, -404.1775)
  line L138 (-202.8825, -404.1775) -> (-174.3075, -404.1775)
  line L139 (-174.3075, -404.1775) -> (-174.3075, -432.7525)
  line L140 (-140.97, -432.7525) -> (-169.545, -432.7525)
  line L141 (-169.545, -432.7525) -> (-169.545, -404.1775)
  line L142 (-169.545, -404.1775) -> (-140.97, -404.1775)
  line L143 (-140.97, -404.1775) -> (-140.97, -432.7525)
  line L144 (-107.6325, -432.7525) -> (-136.2075, -432.7525)
  line L145 (-136.2075, -432.7525) -> (-136.2075, -404.1775)
  line L146 (-136.2075, -404.1775) -> (-107.6325, -404.1775)
  line L147 (-107.6325, -404.1775) -> (-107.6325, -432.7525)
  line L148 (-74.295, -432.7525) -> (-102.87, -432.7525)
  line L149 (-102.87, -432.7525) -> (-102.87, -404.1775)
  line L150 (-102.87, -404.1775) -> (-74.295, -404.1775)
  line L151 (-74.295, -404.1775) -> (-74.295, -432.7525)
  line L152 (-40.9575, -404.1775) -> (-40.9575, -432.7525)
  line L153 (-40.9575, -432.7525) -> (-69.5325, -432.7525)
  line L154 (-69.5325, -432.7525) -> (-69.5325, -404.1775)
  line L155 (-69.5325, -404.1775) -> (-40.9575, -404.1775)
  line L156 (-7.62, -399.415) -> (-36.195, -399.415)
  line L157 (-36.195, -399.415) -> (-36.195, -370.84)
  line L158 (-36.195, -370.84) -> (-7.62, -370.84)
  line L159 (-7.62, -370.84) -> (-7.62, -399.415)
  line L160 (-102.87, -399.415) -> (-102.87, -370.84)
  line L161 (-102.87, -370.84) -> (-74.295, -370.84)
  line L162 (-74.295, -370.84) -> (-74.295, -399.415)
  line L163 (-74.295, -399.415) -> (-102.87, -399.415)
  line L164 (-136.2075, -399.415) -> (-136.2075, -370.84)
  line L165 (-136.2075, -370.84) -> (-107.6325, -370.84)
  line L166 (-107.6325, -370.84) -> (-107.6325, -399.415)
  line L167 (-107.6325, -399.415) -> (-136.2075, -399.415)
  line L168 (-169.545, -399.415) -> (-169.545, -370.84)
  line L169 (-169.545, -370.84) -> (-140.97, -370.84)
  line L170 (-140.97, -370.84) -> (-140.97, -399.415)
  line L171 (-140.97, -399.415) -> (-169.545, -399.415)
  line L172 (-202.8825, -399.415) -> (-202.8825, -370.84)
  line L173 (-202.8825, -370.84) -> (-174.3075, -370.84)
  line L174 (-174.3075, -370.84) -> (-174.3075, -399.415)
  line L175 (-174.3075, -399.415) -> (-202.8825, -399.415)
  line L176 (-236.22, -399.415) -> (-236.22, -370.84)
  line L177 (-236.22, -370.84) -> (-207.645, -370.84)
  line L178 (-207.645, -370.84) -> (-207.645, -399.415)
  line L179 (-207.645, -399.415) -> (-236.22, -399.415)
  line L180 (-269.5575, -399.415) -> (-269.5575, -370.84)
  line L181 (-269.5575, -370.84) -> (-240.9825, -370.84)
  line L182 (-240.9825, -370.84) -> (-240.9825, -399.415)
  line L183 (-240.9825, -399.415) -> (-269.5575, -399.415)
  line L184 (-302.895, -399.415) -> (-302.895, -370.84)
  line L185 (-302.895, -370.84) -> (-274.32, -370.84)
  line L186 (-274.32, -370.84) -> (-274.32, -399.415)
  line L187 (-274.32, -399.415) -> (-302.895, -399.415)
  line L188 (-336.2325, -399.415) -> (-336.2325, -370.84)
  line L189 (-336.2325, -370.84) -> (-307.6575, -370.84)
  line L190 (-307.6575, -370.84) -> (-307.6575, -399.415)
  line L191 (-307.6575, -399.415) -> (-336.2325, -399.415)
  line L192 (-369.57, -399.415) -> (-369.57, -370.84)
  line L193 (-369.57, -370.84) -> (-340.995, -370.84)
  line L194 (-340.995, -370.84) -> (-340.995, -399.415)
  line L195 (-340.995, -399.415) -> (-369.57, -399.415)
  line L196 (-36.195, -432.7525) -> (-36.195, -404.1775)
  line L197 (-36.195, -404.1775) -> (-7.62, -404.1775)
  line L198 (-7.62, -404.1775) -> (-7.62, -432.7525)
  line L199 (-7.62, -432.7525) -> (-36.195, -432.7525)
  line L200 (-402.9075, -432.7525) -> (-402.9075, -404.1775)
  line L201 (-402.9075, -404.1775) -> (-374.3325, -404.1775)
  line L202 (-374.3325, -404.1775) -> (-374.3325, -432.7525)
  line L203 (-374.3325, -432.7525) -> (-402.9075, -432.7525)
  line L204 (-369.57, -432.7525) -> (-369.57, -404.1775)
  line L205 (-369.57, -404.1775) -> (-340.995, -404.1775)
  line L206 (-340.995, -404.1775) -> (-340.995, -432.7525)
  line L207 (-340.995, -432.7525) -> (-369.57, -432.7525)
  line L208 (-307.6575, -432.7525) -> (-336.2325, -432.7525)
  line L209 (-336.2325, -432.7525) -> (-336.2325, -404.1775)
  line L210 (-336.2325, -404.1775) -> (-307.6575, -404.1775)
  line L211 (-307.6575, -404.1775) -> (-307.6575, -432.7525)
  line L212 (-274.32, -432.7525) -> (-302.895, -432.7525)
  line L213 (-302.895, -432.7525) -> (-302.895, -404.1775)
  line L214 (-302.895, -404.1775) -> (-274.32, -404.1775)
  line L215 (-274.32, -404.1775) -> (-274.32, -432.7525)
  line L216 (-240.9825, -432.7525) -> (-269.5575, -432.7525)
  line L217 (-269.5575, -432.7525) -> (-269.5575, -404.1775)
  line L218 (-269.5575, -404.1775) -> (-240.9825, -404.1775)
  line L219 (-240.9825, -404.1775) -> (-240.9825, -432.7525)
  line L220 (-7.62, -304.165) -> (-7.62, -332.74)
  line L221 (-7.62, -332.74) -> (-36.195, -332.74)
  line L222 (-36.195, -332.74) -> (-36.195, -304.165)
  line L223 (-36.195, -304.165) -> (-7.62, -304.165)
  line L224 (-7.62, -337.5025) -> (-7.62, -366.0775)
  line L225 (-7.62, -366.0775) -> (-36.195, -366.0775)
  line L226 (-36.195, -366.0775) -> (-36.195, -337.5025)
  line L227 (-36.195, -337.5025) -> (-7.62, -337.5025)
  line L228 (-7.62, -270.8275) -> (-7.62, -299.4025)
  line L229 (-7.62, -299.4025) -> (-36.195, -299.4025)
  line L230 (-36.195, -299.4025) -> (-36.195, -270.8275)
  line L231 (-36.195, -270.8275) -> (-7.62, -270.8275)
  line L232 (-7.62, -237.49) -> (-7.62, -266.065)
  line L233 (-7.62, -266.065) -> (-36.195, -266.065)
  line L234 (-36.195, -266.065) -> (-36.195, -237.49)
  line L235 (-36.195, -237.49) -> (-7.62, -237.49)
  line L236 (-7.62, -204.1525) -> (-7.62, -232.7275)
  line L237 (-7.62, -232.7275) -> (-36.195, -232.7275)
  line L238 (-36.195, -232.7275) -> (-36.195, -204.1525)
  line L239 (-36.195, -204.1525) -> (-7.62, -204.1525)
  line L240 (-7.62, -170.815) -> (-7.62, -199.39)
  line L241 (-7.62, -199.39) -> (-36.195, -199.39)
  line L242 (-36.195, -199.39) -> (-36.195, -170.815)
  line L243 (-36.195, -170.815) -> (-7.62, -170.815)
  line L244 (-7.62, -137.4775) -> (-7.62, -166.0525)
  line L245 (-7.62, -166.0525) -> (-36.195, -166.0525)
  line L246 (-36.195, -166.0525) -> (-36.195, -137.4775)
  line L247 (-36.195, -137.4775) -> (-7.62, -137.4775)
  line L248 (-69.5325, -332.74) -> (-69.5325, -304.165)
  line L249 (-69.5325, -304.165) -> (-40.9575, -304.165)
  line L250 (-40.9575, -304.165) -> (-40.9575, -332.74)
  line L251 (-40.9575, -332.74) -> (-69.5325, -332.74)
  line L252 (-102.87, -332.74) -> (-102.87, -304.165)
  line L253 (-102.87, -304.165) -> (-74.295, -304.165)
  line L254 (-74.295, -304.165) -> (-74.295, -332.74)
  line L255 (-74.295, -332.74) -> (-102.87, -332.74)
  line L256 (-136.2075, -332.74) -> (-136.2075, -304.165)
  line L257 (-136.2075, -304.165) -> (-107.6325, -304.165)
  line L258 (-107.6325, -304.165) -> (-107.6325, -332.74)
  line L259 (-107.6325, -332.74) -> (-136.2075, -332.74)
  line L260 (-169.545, -332.74) -> (-169.545, -304.165)
  line L261 (-169.545, -304.165) -> (-140.97, -304.165)
  line L262 (-140.97, -304.165) -> (-140.97, -332.74)
  line L263 (-140.97, -332.74) -> (-169.545, -332.74)
  line L264 (-202.8825, -332.74) -> (-202.8825, -304.165)
  line L265 (-202.8825, -304.165) -> (-174.3075, -304.165)
  line L266 (-174.3075, -304.165) -> (-174.3075, -332.74)
  line L267 (-174.3075, -332.74) -> (-202.8825, -332.74)
  line L268 (-236.22, -332.74) -> (-236.22, -304.165)
  line L269 (-236.22, -304.165) -> (-207.645, -304.165)
  line L270 (-207.645, -304.165) -> (-207.645, -332.74)
  line L271 (-207.645, -332.74) -> (-236.22, -332.74)
  line L272 (-269.5575, -332.74) -> (-269.5575, -304.165)
  line L273 (-269.5575, -304.165) -> (-240.9825, -304.165)
  line L274 (-240.9825, -304.165) -> (-240.9825, -332.74)
  line L275 (-240.9825, -332.74) -> (-269.5575, -332.74)
  line L276 (-302.895, -332.74) -> (-302.895, -304.165)
  line L277 (-302.895, -304.165) -> (-274.32, -304.165)
  line L278 (-274.32, -304.165) -> (-274.32, -332.74)
  line L279 (-274.32, -332.74) -> (-302.895, -332.74)
  line L280 (-336.2325, -332.74) -> (-336.2325, -304.165)
  line L281 (-336.2325, -304.165) -> (-307.6575, -304.165)
  line L282 (-307.6575, -304.165) -> (-307.6575, -332.74)
  line L283 (-307.6575, -332.74) -> (-336.2325, -332.74)
  line L284 (-369.57, -332.74) -> (-369.57, -304.165)
  line L285 (-369.57, -304.165) -> (-340.995, -304.165)
  line L286 (-340.995, -304.165) -> (-340.995, -332.74)
  line L287 (-340.995, -332.74) -> (-369.57, -332.74)
  line L288 (-69.5325, -366.0775) -> (-69.5325, -337.5025)
  line L289 (-69.5325, -337.5025) -> (-40.9575, -337.5025)
  line L290 (-40.9575, -337.5025) -> (-40.9575, -366.0775)
  line L291 (-40.9575, -366.0775) -> (-69.5325, -366.0775)